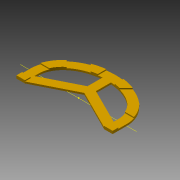
# Autodesk Inventor part: Laseraufbau
Saved by Autodesk Inventor 2014 (Build 180170000, 170)
## iProperties
Created: 2013-12-10
Part Number: Laseraufbau
Material: Generisch
Document SubType Name: Modeling
Designer: Juri
Density: 1 g/cm^3
Appearance: Vorgabe
Author: Juri
Autodesk Inventor part; units mm, degrees
ref_plane "YZ Plane" through (0, 0, 0) normal (1, 0, 0) x (0, 1, 0)
ref_plane "XZ Plane" through (0, 0, 0) normal (0, 1, 0) x (-1, 0, 0)
ref_plane "XY Plane" through (0, 0, 0) normal (0, 0, 1) x (1, 0, 0)
sketch "Skizze1" plane through (0, 0, 0) normal (1, 0, 0) x (0, 1, 0)
  point P0 (0, 0)
sketch "Skizze2" plane through (0, 0, 0) normal (0, 0, 1) x (1, 0, 0)
  line L0 (0, 0) -> (0, 50)
  ellipse E0 centre (0, 0) end of major axis (0, 50) minor radius 70
  ellipse E1 centre (0, 0) end of major axis (85, 0) minor radius 65
  point P0 (0, 65)
  dimension "d3" = 70
  dimension "d4" = 85
  dimension "d1" = 50
  dimension "d5" = 15
  constraints: 3 vertical, 2 coincident, 2 end point, 2 vertical alignment, 4 other
  measures "d1" distance of L0.start L0.end
  measures "d5" distance of L0.end point (0, 65)
extrude "Extrusion1" add sketch "Skizze2" along normal blind 5
sketch "Skizze4" plane through (0, 0, 5) normal (0, 0, 1) x (1, 0, 0)
  line L0 (-138.5421, 0) -> (141.5539, 0)
  line L1 (141.5539, 0) -> (141.5539, -100.2494)
  line L2 (141.5539, -100.2494) -> (-138.5421, -100.2494)
  line L3 (-138.5421, -100.2494) -> (-138.5421, 0)
  constraints: 8 end point, 2 parallel, 1 horizontal, 1 perpendicular
extrude "Extrusion3" cut sketch "Skizze4" against normal blind 5
sketch "Skizze5" plane through (0, 0, 5) normal (0, 0, 1) x (1, 0, 0)
  line L0 (-85, 0) -> (-70, 0)
  line L1 (-70, 0) -> (-70, -25)
  line L2 (-70, -25) -> (-85, -25)
  line L3 (-85, -25) -> (-85, 0)
  line L4 (70, 0) -> (85, 0)
  line L5 (85, 0) -> (85, -25)
  line L6 (85, -25) -> (70, -25)
  line L7 (70, -25) -> (70, 0)
  dimension "d13" = 25
  dimension "d14" = 25
  constraints: 16 end point, 4 parallel, 2 horizontal, 2 perpendicular
  measures "d13" distance of L2.end L0.start
  measures "d14" distance of L4.end L5.end
extrude "Extrusion4" add sketch "Skizze5" against normal blind 5
sketch "Skizze7" plane through (0, 0, 5) normal (0, 0, 1) x (1, 0, 0)
  line L0 (14.5161, 65.7113) -> (16.129, 65.7113)
  line L1 (16.129, 65.7113) -> (16.129, 66.0339)
  line L2 (16.129, 66.0339) -> (14.5161, 66.0339)
  line L3 (14.5161, 66.0339) -> (14.5161, 65.7113)
  line L4 (-15, 28.2919) -> (15, 28.2919)
  line L5 (15, 28.2919) -> (15, 68.6145)
  line L6 (15, 68.6145) -> (-15, 68.6145)
  line L7 (-15, 68.6145) -> (-15, 28.2919)
  line L8 (-70, -25) -> (-85, -25) projected
  line L9 (-85, -25) -> (-85, 0) projected
  ellipse E0 centre (0, 0) end of major axis (-85, 0) minor radius 65 (85, 0) -> (-85, 0) ccw projected
  line L10 (85, 0) -> (85, -25) projected
  line L11 (85, -25) -> (70, -25) projected
  line L12 (70, -25) -> (70, 0) projected
  ellipse E1 centre (0, 0) end of major axis (-70, 0) minor radius 50 (70, 0) -> (-70, 0) ccw projected
  line L13 (-70, 0) -> (-70, -25) projected
  line L14 (0, -43.7229) -> (0, 87.3374) projected
  dimension "d20" = 30
  constraints: 16 end point, 4 parallel, 2 horizontal, 2 perpendicular, 3 other
  measures "d20" distance of L5.end L6.end
extrude "Extrusion5" cut sketch "Skizze7" against normal blind 2 contours L3 L2 L5 L0 | L0 L5 E0 L14 L6 L2 L3 | L5 E1 L14 E0 | L5 L4 L14 E1 | L14 E1 L7 E0 | E0 L7 L6 L14 | L14 L4 L7 E1
sketch "Skizze8" plane through (0, 0, 5) normal (0, 0, 1) x (1, 0, 0)
  ellipse E0 centre (0, 0) end of major axis (-85, 0) minor radius 65 (85, 0) -> (15, 63.9799) ccw projected
  line L0 (0, 0) -> (49.3064, 49.3064) construction
  line L1 (-121.351, 0) -> (133.1061, 0) construction
  line L2 (76.2939, 97.5071) -> (19.9385, 41.1517)
  line L3 (19.9385, 41.1517) -> (41.1517, 19.9385)
  line L4 (41.1517, 19.9385) -> (92.1355, 70.9223)
  line L5 (76.2939, 97.5071) -> (92.1355, 70.9223)
  dimension "d23" = 45
  dimension "d24" = 30
  constraints: 10 end point, 2 parallel, 1 perpendicular, 2 other
  measures "d23" angle of L1 L0
  measures "d24" distance of L2.end L3.end
extrude "Extrusion6" cut sketch "Skizze8" against normal blind 2
sketch "Skizze9" plane through (0, 0, 5) normal (0, 0, 1) x (1, 0, 0)
  line L0 (52.5724, 15) -> (140.4, 15)
  line L1 (140.4, 15) -> (140.4, -15)
  line L2 (140.4, -15) -> (52.5724, -15)
  line L3 (52.5724, -15) -> (52.5724, 15)
  line L4 (-125.4, 0) -> (157.4, 0) projected
  dimension "d27" = 30
  constraints: 8 end point, 2 parallel, 1 horizontal, 1 perpendicular, 1 other
  measures "d27" distance of L0.end L1.end
extrude "Extrusion7" cut sketch "Skizze9" against normal blind 2
sketch "Skizze10" plane through (0, 0, 5) normal (0, 0, 1) x (1, 0, 0)
  ellipse E0 centre (0, 0) end of major axis (-70, 0) minor radius 50 (-15, 48.8386) -> (-70, 0) ccw projected
  line L0 (0, 0) -> (-45.6382, 45.6382) construction
  line L1 (-155, 0) -> (125, 0) projected
  line L2 (-28.1942, 6.981) -> (-6.981, 28.1942)
  line L3 (-6.981, 28.1942) -> (-56.587, 77.8002)
  line L4 (-56.587, 77.8002) -> (-77.8002, 56.587)
  line L5 (-28.1942, 6.981) -> (-77.8002, 56.587)
  dimension "d30" = 45
  dimension "d31" = 30
  constraints: 10 end point, 1 parallel, 1 perpendicular, 2 other
  measures "d30" angle of L1 L0
  measures "d31" distance between parallel lines of L3 L5
extrude "Extrusion8" cut sketch "Skizze10" against normal blind 2
sketch "Skizze11" plane through (0, 0, 5) normal (0, 0, 1) x (1, 0, 0)
  ellipse E0 centre (0, 0) end of major axis (-70, 0) minor radius 50 (-53.4768, 32.2636) -> (-70, 0) ccw projected
  line L0 (-171.6, -15) -> (-171.6, 15)
  line L1 (-171.6, 15) -> (-38.4, 15)
  line L2 (-38.4, 15) -> (-38.4, -15)
  line L3 (-38.4, -15) -> (-171.6, -15)
  line L4 (-188.6, 0) -> (130.6, 0) projected
  dimension "d34" = 30
  constraints: 8 end point, 2 parallel, 1 perpendicular, 1 vertical, 2 other
  measures "d34" distance between parallel lines of L3 L1
extrude "Extrusion9" cut sketch "Skizze11" against normal blind 2
sketch "Skizze12" plane through (0, 0, 3) normal (0, 0, 1) x (1, 0, 0)
  ellipse E0 centre (0, 0) end of major axis (-70, 0) minor radius 50 (15, 48.8386) -> (-15, 48.8386) ccw projected
  line L0 (-15, 48.8386) -> (-15, 63.9799) projected
  line L1 (-7.5, 49.7122) -> (-7.5, 23.0205)
  line L2 (0, -43) -> (0, 83) construction
  line L3 (7.5, 49.7122) -> (7.5, 23.0205)
  line L4 (-7.5, 23.0205) -> (-70, -8.2295)
  line L5 (-70, 0) -> (-70, -15) construction
  line L6 (7.5, 23.0205) -> (70, -8.2295)
  line L7 (70, -15) -> (70, 0) construction
  line L8 (-70, -8.2295) -> (-70, -25)
  line L9 (70, -25) -> (70, -8.2295)
  line L10 (-7.5, 49.7122) -> (0, 53)
  line L11 (0, 53) -> (7.5, 49.7122)
  line L12 (0, 10) -> (-70, -25)
  line L13 (0, 10) -> (70, -25)
  dimension "d37" = 15
  dimension "d41" = 53
  dimension "d43" = 15
  dimension "d44" = 15
  dimension "d45" = 10
  constraints: 20 end point, 4 parallel, 4 point on line, 1 collinear, 1 vertical, 4 other
  measures "d37" distance between parallel lines of L3 L1
  measures "d41" distance of point (0, 0) L10.end
  measures "d43" distance between parallel lines of L12 L4
  measures "d44" distance between parallel lines of L6 L13
  measures "d45" distance of point (0, 0) L12.start
extrude "Extrusion10" add sketch "Skizze12" against normal blind 3
